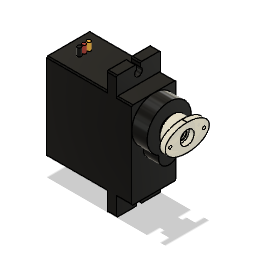
Door Assmebly (Autodesk Fusion 360 archive; units mm, degrees)
design "Micro Servo"
Autodesk Fusion 360 part; units mm, degrees
sketch "Sketch1" plane through (0, 0, 0) normal (0, 1, 0) x (1, 0, 0) in component "servo"
  line L0 (-0.0173, 0.0075) -> (22.1827, 0.0075)
  line L1 (22.1827, 0.0075) -> (22.1827, -12.1925)
  line L2 (22.1827, -12.1925) -> (-0.0173, -12.1925)
  line L3 (-0.0173, -12.1925) -> (-0.0173, 0.0075)
  line L4 (-0.0173, 0.0075) -> (22.1827, -12.1925) construction
  line L5 (22.1827, 0.0075) -> (-0.0173, -12.1925) construction
  point P0 (11.0827, -6.0925)
  dimension "d3" = 12.2
  dimension "d4" = 22.2
  constraint perpendicular L0 L1
  constraint parallel L0 L2
  constraint parallel L1 L3
  constraint horizontal L0
  constraint coincident L4 P0
  constraint coincident L5 P0
  measures "d3" distance of L0.end L1.end
  measures "d4" distance of L1.end L2.end
extrude "Extrude1" add sketch "Sketch1" along normal blind 22.62 in component "servo"
sketch "Sketch2" plane through (22.1827, 0, 0) normal (1, 0, 0) x (0, 0, -1) in component "servo"
  line L0 (-12.1925, 0) -> (0.0075, 0)
  line L1 (0.0075, 0) -> (0.0075, 22.62)
  line L2 (0.0075, 22.62) -> (-12.1925, 22.62)
  line L3 (-12.1925, 22.62) -> (-12.1925, 0)
  circle A0 centre (-5.7425, 16.87) radius 5.75
  dimension "d7" = 11.5
  constraint tangent L1 A0
  constraint tangent L2 A0
  measures "d7" diameter of A0
move_face "OffsetFaces1" offset -0.7 1 faces at (14.7827, 7.54, 12.1925) in component "servo"
extrude "Extrude2" add sketch "Sketch2" along normal blind 4 contours A0 in component "servo"
sketch "Sketch3" plane through (22.1827, 0, 0) normal (1, 0, 0) x (0, 0, -1) in component "servo"
  arc A0 (-11.4925, 16.87) -> (0.0075, 16.87) centre (-5.7425, 16.87) ccw
  line L0 (-11.4925, 16.87) -> (-11.4925, 0)
  line L1 (-11.4925, 0) -> (0.0075, 0)
  line L2 (0.0075, 0) -> (0.0075, 16.87)
  circle A1 centre (-5.7425, 11.12) radius 2.75
  dimension "d11" = 5.5
  constraint midpoint A0 A1.centre
  measures "d11" diameter of A1
extrude "Extrude3" add sketch "Sketch3" along normal blind 4 contours A0 A1 picked at (-5.7857, 10.2135) in component "servo"
sketch "Sketch4" plane through (26.1827, 0, 0) normal (1, 0, 0) x (0, 0, -1) in component "servo"
  arc A0 (-3.0723, 11.7776) -> (-8.4127, 11.7776) centre (-5.7425, 16.87) ccw
  arc A1 (-8.4127, 11.7776) -> (-3.0723, 11.7776) centre (-5.7425, 11.12) ccw
  circle A2 centre (-5.7425, 16.87) radius 2.4
  dimension "d14" = 4.8
  constraint concentric A0 A2
  measures "d14" diameter of A2
extrude "Extrude4" add sketch "Sketch4" along normal blind 3 contours A2 in component "servo"
sketch "Sketch5" plane through (0, 22.62, 0) normal (0, 1, 0) x (-1, 0, 0) in component "servo"
  line L0 (0.0173, 11.4925) -> (-22.1827, 11.4925)
  line L1 (-22.1827, 11.4925) -> (-22.1827, 5.7425)
  line L2 (-22.1827, 5.7425) -> (-22.1827, -0.0075)
  line L3 (-22.1827, -0.0075) -> (0.0173, -0.0075)
  line L4 (0.0173, -0.0075) -> (0.0173, 11.4925)
  line L5 (-18.1827, 0) -> (-15.7827, 0)
  line L6 (-15.7827, 0) -> (-15.7827, 11.485)
  line L7 (-15.7827, 11.485) -> (-18.1827, 11.485)
  line L8 (-18.1827, 11.485) -> (-18.1827, 0)
  line L9 (-18.1827, 0) -> (-15.7827, 11.485) construction
  line L10 (-15.7827, 0) -> (-18.1827, 11.485) construction
  line L11 (-22.1827, 11.4925) -> (0.0173, 11.4925)
  line L12 (0.0173, 11.4925) -> (0.0173, -0.0075)
  line L13 (0.0173, -0.0075) -> (-22.1827, -0.0075)
  line L14 (-22.1827, -0.0075) -> (-22.1827, 11.4925)
  point P0 (-16.9827, 5.7425)
  dimension "d17" = 2.4
  dimension "d18" = 4
  constraint perpendicular L5 L6
  constraint parallel L5 L7
  constraint parallel L6 L8
  constraint horizontal L5
  constraint coincident L9 P0
  constraint coincident L10 P0
  measures "d17" distance of L6.end L7.end
  measures "d18" distance of L1.end L8
extrude "Extrude5" add sketch "Sketch5" along normal blind 4.7 contours L5 L6 L7 L8 in component "servo"
sketch "Sketch6" plane through (0, 27.32, 0) normal (0, 1, 0) x (-1, 0, 0) in component "servo"
  line L0 (-18.1827, 11.485) -> (-18.1827, 0)
  line L1 (-18.1827, 0) -> (-15.7827, 0)
  line L2 (-15.7827, 0) -> (-15.7827, 11.485)
  line L3 (-15.7827, 11.485) -> (-18.1827, 11.485)
  line L4 (-22.1827, 11.4925) -> (0.0173, 11.4925)
  line L5 (0.0173, 11.4925) -> (0.0173, -0.0075)
  line L6 (0.0173, -0.0075) -> (-22.1827, -0.0075)
  line L7 (-22.1827, -0.0075) -> (-22.1827, 11.4925)
  line L8 (-22.1827, -0.0075) -> (0.0173, -0.0075)
  line L9 (0.0173, -0.0075) -> (-22.1827, -0.0075)
  line L10 (-15.7827, 11.485) -> (-18.1827, 11.485)
  line L11 (-18.1827, 11.485) -> (-15.7827, 11.485)
  line L12 (-18.1827, 0) -> (-15.7827, 0)
  line L13 (-15.7827, 0) -> (-18.1827, 0)
sketch "Sketch7" plane through (0, 0, 0) normal (0, -1, 0) x (1, 0, 0) in component "servo"
  line L0 (22.1827, 11.4925) -> (-0.0173, 11.4925)
  line L1 (-0.0173, 11.4925) -> (-0.0173, -0.0075)
  line L2 (-0.0173, -0.0075) -> (22.1827, -0.0075)
  line L3 (22.1827, -0.0075) -> (22.1827, 11.4925)
  line L4 (18.1827, 0) -> (15.7827, 0)
  line L5 (15.7827, 0) -> (15.7827, 11.485)
  line L6 (15.7827, 11.485) -> (18.1827, 11.485)
  line L7 (18.1827, 11.485) -> (18.1827, 0)
  line L8 (18.1827, 0) -> (15.7827, 11.485) construction
  line L9 (15.7827, 0) -> (18.1827, 11.485) construction
  point P0 (16.9827, 5.7425)
  point P1 (16.9827, 5.7425)
  point P2 (18.1827, 0)
  constraint perpendicular L4 L5
  constraint parallel L4 L6
  constraint parallel L5 L7
  constraint horizontal L4
  constraint coincident P2 L4.start
  constraint coincident L8 P1
  constraint coincident L9 P1
  constraint coincident P1 P0
extrude "Extrude6" add sketch "Sketch7" along normal blind 4.7 contours L4 L5 L6 L7 in component "servo"
sketch "Sketch8" plane through (18.1827, 0, 0) normal (1, 0, 0) x (0, 0, -1) in component "servo"
  line L0 (-11.485, 22.62) -> (0, 22.62)
  line L1 (0, 22.62) -> (0, 27.32)
  line L2 (0, 27.32) -> (-11.485, 27.32)
  line L3 (-11.485, 27.32) -> (-11.485, 22.62)
  circle A0 centre (-5.7425, 25.32) radius 1
  line L4 (-5.7425, 27.32) -> (-5.7425, 22.62) construction
  line L5 (-5.2425, 27.32) -> (-5.2425, 26.186)
  line L6 (-6.2425, 27.32) -> (-6.2425, 26.186)
  point P0 (-5.7425, 22.62)
  dimension "d23" = 2
  dimension "d24" = 2
  dimension "d27" = 1
  constraint midpoint L2 L4.start
  constraint coincident P0 L4.end
  constraint coincident A0.centre L4
  constraint coincident L2 L5.start
  constraint coincident A0 L5.end
  constraint perpendicular L2 L5
  constraint coincident L2 L6.start
  constraint coincident A0 L6.end
  constraint perpendicular L2 L6
  measures "d23" diameter of A0
  measures "d24" distance of L2 A0.centre
  measures "d27" distance of L5 L6
extrude "Extrude7" cut sketch "Sketch8" against normal up to surface (2.4 mm away) contours L2 A0 L5 L6 | A0 in component "servo"
sketch "Sketch9" plane through (18.1827, 0, 0) normal (1, 0, 0) x (0, 0, -1) in component "servo"
  line L0 (0, 0) -> (-11.485, 0)
  line L1 (-11.485, 0) -> (-11.485, -4.7)
  line L2 (-11.485, -4.7) -> (0, -4.7)
  line L3 (0, -4.7) -> (0, 0)
  circle A0 centre (-5.7412, -2.7) radius 1
  line L4 (-5.7425, 0) -> (-5.7425, -4.7) construction
  line L5 (-5.2425, -3.5668) -> (-5.2425, -4.7)
  line L6 (-6.2425, -3.5653) -> (-6.2425, -4.7)
  dimension "d30" = 2
  dimension "d31" = 2
  dimension "d33" = 1
  constraint midpoint L0 L4.start
  constraint midpoint L2 L4.end
  constraint coincident A0 L5.start
  constraint coincident L2 L5.end
  constraint perpendicular L2 L5
  constraint coincident A0 L6.start
  constraint coincident L2 L6.end
  constraint perpendicular L2 L6
  measures "d30" diameter of A0
  measures "d31" distance of A0.centre L4.end
  measures "d33" distance of L5 L6
extrude "Extrude8" cut sketch "Sketch9" against normal up to surface (2.4 mm away) contours L2 A0 L5 L6 | A0 in component "servo"
sketch "Sketch10" plane through (0, 0, -0.0075) normal (0, 0, -1) x (-1, 0, 0) in component "servo"
  line L0 (-22.1827, 0) -> (0.0173, 0)
  line L1 (0.0173, 0) -> (0.0173, 22.62)
  line L2 (0.0173, 22.62) -> (-22.1827, 22.62)
  line L3 (-22.1827, 22.62) -> (-22.1827, 16.87)
  line L4 (-22.1827, 16.87) -> (-22.1827, 0)
sketch "Sketch11" plane through (0, 22.62, 0) normal (0, 1, 0) x (-1, 0, 0) in component "servo"
  line L0 (-18.1827, 11.485) -> (-15.7827, 11.485)
  line L1 (-15.7827, 11.485) -> (-15.7827, 0)
  line L2 (-15.7827, 0) -> (-18.1827, 0)
  line L3 (-18.1827, 0) -> (-18.1827, 11.485)
  line L4 (0.0173, 11.4925) -> (-22.1827, 11.4925)
  line L5 (-22.1827, 11.4925) -> (-22.1827, 5.7425)
  line L6 (-22.1827, 5.7425) -> (-22.1827, -0.0075)
  line L7 (-22.1827, -0.0075) -> (0.0173, -0.0075)
  line L8 (0.0173, -0.0075) -> (0.0173, 11.4925)
  line L9 (-3.9827, 4.4925, 0) -> (-3.9827, 4.4925, 2)
  line L10 (0.0173, -0.0075) -> (-22.1827, -0.0075)
  line L11 (-3.9827, 5.7425, 0) -> (-3.9827, 5.7425, 2)
  line L12 (-3.9827, 6.9925, 0) -> (-3.9827, 6.9925, 2)
  dimension "d37" = 4
  dimension "d38" = 4.5
  dimension "d39" = 4.5
pipe "Pipe1" add diameter 1 path "Sketch11" along L9 in component "servo"
pipe "Pipe2" add diameter 1 path "Sketch11" along L11 in component "servo"
pipe "Pipe3" add diameter 1 path "Sketch11" along L12 in component "servo"
sketch "Sketch12" plane through (29.1827, 0, 0) normal (1, 0, 0) x (0, 0, -1) in component "servo"
  circle A0 centre (-5.7425, 16.87) radius 2.4
  circle A1 centre (-5.7425, 16.87) radius 3.45
  dimension "d53" = 6.9
  constraint concentric A0 A1
  measures "d53" diameter of A1
extrude "Extrude9" add sketch "Sketch12" against normal blind 2 in component "servo"
move_face "OffsetFaces2" offset 1.72 1 faces at (29.1827, 16.0878, 6.0495) in component "servo"
sketch "Sketch13" plane through (30.9027, 0, 0) normal (1, 0, 0) x (0, 0, -1) in component "servo"
  circle A0 centre (-5.7425, 16.87) radius 3.45
  ellipse E0 centre (-5.7425, 16.87) end of major axis (0.0075, 16.87) minor radius 3.45
  line L0 (-11.4925, 16.87) -> (0.0075, 16.87)
  line L1 (-5.7425, 13.42) -> (-5.7425, 20.32)
  line L2 (0.0075, 0) -> (0.0075, 22.62)
  point P0 (0.0075, 16.87)
  constraint concentric A0 E0
  constraint perpendicular L0 L2
  constraint coincident E0 L0.start
  constraint coincident E0 P0
  constraint coincident E0 L1.start
  constraint coincident E0 L1.end
extrude "Extrude10" add sketch "Sketch13" against normal blind 1.4 contours A0 E0 L0 | A0 E0 L0 | A0 E0 L0 | A0 E0 L0 in component "servo"
sketch "Sketch14" plane through (30.9027, 0, 0) normal (1, 0, 0) x (0, 0, -1) in component "servo"
  arc A0 (-5.7573, 13.42) -> (-5.7276, 13.42) centre (-5.7425, 16.87) ccw
  ellipse E0 centre (-5.7425, 16.87) end of major axis (0.0075, 16.87) minor radius 3.45 (-5.7276, 13.42) -> (-5.7276, 20.32) ccw
  arc A1 (-5.7276, 20.32) -> (-5.7573, 20.32) centre (-5.7425, 16.87) ccw
  ellipse E1 centre (-5.7425, 16.87) end of major axis (0.0075, 16.87) minor radius 3.45 (-5.7573, 20.32) -> (-5.7573, 13.42) ccw
  circle A2 centre (-1.3212, 16.87) radius 0.4
  circle A3 centre (-10.1636, 16.9081) radius 0.4
  line L0 (-5.7276, 20.32) -> (-5.7573, 13.42) construction
  dimension "d59" = 0.8
  dimension "d60" = 0.8
  constraint coincident A1.start L0.start
  constraint coincident A0.start L0.end
  constraint symmetric A2.centre A3.centre L0
  measures "d59" diameter of A2
  measures "d60" diameter of A3
extrude "Extrude11" cut sketch "Sketch14" against normal up to surface (1.4 mm away) contours A2 in component "servo"
extrude "Extrude12" cut sketch "Sketch14" against normal up to surface (1.4 mm away) contours A3 in component "servo"
sketch "Sketch15" plane through (30.9027, 0, 0) normal (1, 0, 0) x (0, 0, -1) in component "servo"
  circle A0 centre (-10.1636, 16.9081) radius 0.4
  circle A1 centre (-1.3212, 16.87) radius 0.4
  arc A2 (-5.7573, 13.42) -> (-5.7276, 13.42) centre (-5.7425, 16.87) ccw
  ellipse E0 centre (-5.7425, 16.87) end of major axis (0.0075, 16.87) minor radius 3.45 (-5.7276, 13.42) -> (-5.7276, 20.32) ccw
  arc A3 (-5.7276, 20.32) -> (-5.7573, 20.32) centre (-5.7425, 16.87) ccw
  ellipse E1 centre (-5.7425, 16.87) end of major axis (0.0075, 16.87) minor radius 3.45 (-5.7573, 20.32) -> (-5.7573, 13.42) ccw
  circle A4 centre (-5.7425, 16.87) radius 1.8
  dimension "d65" = 3.6
  constraint concentric A2 A4
  measures "d65" diameter of A4
extrude "Extrude13" cut sketch "Sketch15" against normal blind 1.3 contours A4 in component "servo"
sketch "Sketch16" plane through (29.6027, 0, 0) normal (1, 0, 0) x (0, 0, -1) in component "servo"
  circle A0 centre (-5.7425, 16.87) radius 1.8
  circle A1 centre (-5.7425, 16.87) radius 1.225
  dimension "d68" = 2.45
  constraint concentric A0 A1
  measures "d68" diameter of A1
extrude "Extrude14" cut sketch "Sketch16" against normal blind 0.2 contours A1 in component "servo"
sketch "Sketch17" plane through (29.4027, 0, 0) normal (1, 0, 0) x (0, 0, -1) in component "servo"
  circle A0 centre (-5.7425, 16.87) radius 1.225
  circle A1 centre (-5.7425, 16.87) radius 0.85
  dimension "d71" = 1.7
  constraint concentric A0 A1
  measures "d71" diameter of A1
extrude "Extrude15" cut sketch "Sketch17" against normal blind 3 contours A1 in component "servo"
thread "Thread1" "ISO Metric profile 1.6 M1.6x0.35 6H" major diameter 1.668 minor diameter 1.271 pitch 0.35 angle 60 resizes the face on face at (27.4027, 17.2002, 4.9592) in component "servo"
extrude "Extrude16" add 1 faces at (17.3827, -1.5667, 0) along direction (0, 0, -1) up to surface (0.0075 mm away) in component "servo"
extrude "Extrude17" add 1 faces at (16.5827, -1.5667, 11.485) along direction (0, 0, 1) up to surface (0.0075 mm away) in component "servo"
extrude "Extrude18" add 1 faces at (16.5827, 24.1867, 11.485) along direction (0, 0, 1) up to surface (0.0075 mm away) in component "servo"
extrude "Extrude19" add 1 faces at (17.3827, 24.1867, 0) along direction (0, 0, -1) up to surface (0.0075 mm away) in component "servo"
fillet "Fillet1" radius 0.3 16 edges at (7.8827, 22.62, -0.0075) (16.9827, 27.32, -0.0075) (16.9827, 27.32, 5.2425) (16.9827, 27.32, 6.2425) (16.9827, 27.32, 11.4925) (20.1827, 22.62, 11.4925) (20.1827, 22.62, -0.0075) (7.8827, 22.62, 11.4925) (20.1827, 0, -0.0075) (7.8827, 0, -0.0075) (16.9827, -4.7, -0.0075) (16.9827, -4.7, 6.2425) (16.9827, -4.7, 5.2425) (16.9827, -4.7, 11.4925) (20.1827, 0, 11.4925) (7.8827, 0, 11.4925) in component "servo"
component "servo" placed x (1, 0, 0) y (0, 1, 0) z (0, 0, 1) at (0, 0, 0)

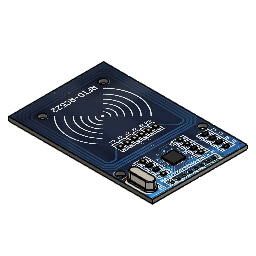
design "RFID"
Autodesk Fusion 360 part; units mm, degrees
sketch "Sketch1" plane through (0, 0, 0) normal (0, 1, 0) x (1, 0, 0) in component "Base"
  line L0 (0, 0) -> (60, 0)
  line L1 (60, 0) -> (60, -39.6)
  line L2 (60, -39.6) -> (0, -39.6)
  line L3 (0, -39.6) -> (0, 0)
  circle A0 centre (7.05, -32.45) radius 1.55
  line L4 (5.5, -34) -> (0, -34) construction
  line L5 (5.5, -34) -> (5.5, -39.6) construction
  circle A1 centre (7.05, -7.15) radius 1.55
  line L6 (5.5, 0) -> (5.5, -5.6) construction
  line L7 (5.5, -5.6) -> (0, -5.6) construction
  line L8 (0, -1.0831) -> (42.4499, -1) construction
  line L9 (42.4499, -1) -> (42.4499, 0) construction
  circle A2 centre (43.9999, -2.547) radius 1.55
  line L10 (0, -38.6) -> (42.45, -38.6) construction
  line L11 (42.45, -38.6) -> (42.45, -39.6) construction
  circle A3 centre (44, -37.05) radius 1.55
  line L12 (49.05, -33.9) -> (55.45, -33.9)
  line L13 (57.6, -36.05) -> (57.6, -36.15)
  line L14 (55.45, -38.3) -> (49.05, -38.3)
  line L15 (46.9, -36.15) -> (46.9, -36.05)
  arc A4 (49.05, -33.9) -> (46.9, -36.05) centre (49.05, -36.05) ccw
  arc A5 (46.9, -36.15) -> (49.05, -38.3) centre (49.05, -36.15) ccw
  arc A6 (57.6, -36.05) -> (55.45, -33.9) centre (55.45, -36.05) ccw
  arc A7 (55.45, -38.3) -> (57.6, -36.15) centre (55.45, -36.15) ccw
  line L16 (55.45, -37.85) -> (49.05, -37.85)
  arc A8 (47.35, -36.15) -> (49.05, -37.85) centre (49.05, -36.15) ccw
  line L17 (47.35, -36.15) -> (47.35, -36.05)
  arc A9 (49.05, -34.35) -> (47.35, -36.05) centre (49.05, -36.05) ccw
  line L18 (49.05, -34.35) -> (55.45, -34.35)
  arc A10 (57.15, -36.05) -> (55.45, -34.35) centre (55.45, -36.05) ccw
  line L19 (57.15, -36.05) -> (57.15, -36.15)
  arc A11 (55.45, -37.85) -> (57.15, -36.15) centre (55.45, -36.15) ccw
  line L20 (46.9, -38.3) -> (46.9, -39.6) construction
  line L21 (57.6, -33.9) -> (60, -33.9) construction
  line L22 (58, -39.6) -> (58, -29.2) construction
  line L23 (58, -29.2) -> (60, -29.2) construction
  circle A12 centre (58, -29.2) radius 0.525
  circle A13 centre (58, -26.7) radius 0.525
  circle A14 centre (58, -24.2) radius 0.525
  circle A15 centre (58, -21.7) radius 0.525
  circle A16 centre (58, -19.2) radius 0.525
  circle A17 centre (58, -16.7) radius 0.525
  circle A18 centre (58, -14.2) radius 0.525
  circle A19 centre (58, -11.7) radius 0.525
  point P0 (46.9, -33.9)
  point P1 (57.6, -33.9)
  point P2 (46.9, -38.3)
  dimension "d1" = 60
  dimension "d2" = 39.6
  dimension "d5" = 3.1
  dimension "d8" = 5.6
  dimension "d9" = 5.5
  dimension "d10" = 3.1
  dimension "d11" = 5.6
  dimension "d12" = 5.5
  dimension "d13" = 42.45
  dimension "d14" = 1
  dimension "d15" = 3.1
  dimension "d16" = 42.45
  dimension "d17" = 1
  dimension "d18" = 3.1
  dimension "d19" = 10.7
  dimension "d20" = 4.4
  dimension "d23" = 0.45
  dimension "d24" = 2.15
  dimension "d25" = 2.4
  dimension "d26" = 1.3
  dimension "d27" = 10.4
  dimension "d28" = 2
  dimension "d29" = 1.05
  dimension "d32" = 0
  dimension "d33" = 2.5
  constraint horizontal L0
  constraint vertical L1
  constraint horizontal L2
  constraint vertical L3
  constraint coincident L0.start L3.end
  constraint coincident L3 L4.end
  constraint perpendicular L3 L4
  constraint coincident L2 L5.end
  constraint perpendicular L2 L5
  constraint coincident L0 L6.start
  constraint tangent A1 L6
  constraint coincident L3 L7.end
  constraint perpendicular L3 L7
  constraint tangent A1 L7
  constraint coincident L3 L8.start
  constraint coincident L0 L9.end
  constraint perpendicular L0 L9
  constraint tangent L8 A2
  constraint tangent L9 A2
  constraint coincident L3 L10.start
  constraint coincident L2 L11.end
  constraint perpendicular L2 L11
  constraint tangent L11 A3
  constraint tangent L10 A3
  constraint coincident P0 L12
  constraint coincident P0 L15
  constraint tangent L12 A4
  constraint tangent L15 A4
  constraint coincident P2 L14
  constraint coincident P2 L15
  constraint tangent L14 A5
  constraint tangent L15 A5
  constraint equal A4 A5
  constraint coincident P1 L12
  constraint coincident P1 L13
  constraint tangent L12 A6
  constraint tangent L13 A6
  constraint equal A4 A6
  constraint tangent L13 A7
  constraint tangent L14 A7
  constraint equal A4 A7
  constraint coincident P2 L20.start
  constraint coincident L2 L20.end
  constraint perpendicular L2 L20
  constraint coincident P1 L21.start
  constraint coincident L1 L21.end
  constraint perpendicular L1 L21
  constraint coincident L2 L22.start
  constraint coincident L1 L23.end
  constraint perpendicular L1 L23
  constraint coincident L22.end L23.start
  measures "d1" distance of L0.start L0.end
  measures "d2" distance of L0.start L2.end
  measures "d5" diameter of A0
  measures "d8" distance of L4.start L5.end
  measures "d9" distance of L4.start L4.end
  measures "d10" diameter of A1
  measures "d11" distance of L6.start L6.end
  measures "d12" distance of L6.end L7.end
  measures "d13" distance of L8.start L8.end
  measures "d14" distance of L8.end L9.end
  measures "d15" diameter of A2
  measures "d16" distance of L10.start L10.end
  measures "d17" distance of L10.end L11.end
  measures "d18" diameter of A3
  measures "d19" distance of P0 P1
  measures "d20" distance of P0 P2
  measures "d24" radius of A4
  measures "d25" distance of P1 L21.end
  measures "d26" distance of P2 L20.end
  measures "d27" distance of L22.start L22.end
  measures "d28" distance of L22.end L23.end
  measures "d29" diameter of A12
extrude "Extrude1" add sketch "Sketch1" against normal blind 1.6 contours L0 L1 L2 L3 | L12 L13 L14 L15 A4 A5 A6 A7 | L16 A8 L17 A9 L18 A10 L19 A11 makes body 1 in component "Base"
extrude "Extrude2" add sketch "Sketch1" along normal blind 0.7 separate body contours L12 L13 L14 L15 A4 A5 A6 A7 | L16 A8 L17 A9 L18 A10 L19 A11 makes body 2 in component "Base"
extrude "Extrude3" add sketch "Sketch1" along normal blind 3.55 separate body contours L16 A8 L17 A9 L18 A10 L19 A11 makes body 3 in component "Base"
fillet "Fillet1" radius 0.25 8 edges at (47.35, 3.55, 36.1) (47.8479, 3.55, 37.3521) (52.25, 3.55, 37.85) (56.6521, 3.55, 37.3521) (57.15, 3.55, 36.1) (56.6521, 3.55, 34.8479) (52.25, 3.55, 34.35) (47.8479, 3.55, 34.8479) on bodies 3 in component "Base"
combine "Combine1" operation add target body 2 tool bodies 3 in component "Base"
sketch "Sketch2" plane through (0, 0, 0) normal (0, 1, 0) x (1, 0, 0) in component "Base"
  line L0 (47.0522, -4.3477) -> (48.2693, -4.3477)
  line L1 (48.2693, -4.3477) -> (48.2693, -6.0785)
  line L2 (48.2693, -6.0785) -> (47.0522, -6.0785)
  line L3 (47.0522, -6.0785) -> (47.0522, -4.3477)
  line L4 (49.9732, -4.226) -> (51.1904, -4.226)
  line L5 (51.1904, -4.226) -> (51.1904, -5.9568)
  line L6 (51.1904, -5.9568) -> (49.9732, -5.9568)
  line L7 (49.9732, -5.9568) -> (49.9732, -4.226)
  line L8 (52.7686, -4.3029) -> (53.9858, -4.3029)
  line L9 (53.9858, -4.3029) -> (53.9858, -6.0337)
  line L10 (53.9858, -6.0337) -> (52.7686, -6.0337)
  line L11 (52.7686, -6.0337) -> (52.7686, -4.3029)
  line L12 (55.7501, -4.3253) -> (56.9673, -4.3253)
  line L13 (56.9673, -4.3253) -> (56.9673, -6.0561)
  line L14 (56.9673, -6.0561) -> (55.7501, -6.0561)
  line L15 (55.7501, -6.0561) -> (55.7501, -4.3253)
  line L16 (43.8016, -11.8351) -> (45.0188, -11.8351)
  line L17 (45.0188, -11.8351) -> (45.0188, -13.0727)
  line L18 (45.0188, -13.0727) -> (43.8016, -13.0727)
  line L19 (43.8016, -13.0727) -> (43.8016, -11.8351)
  line L20 (46.8056, -11.8576) -> (48.0227, -11.8576)
  line L21 (48.0227, -11.8576) -> (48.0227, -13.0951)
  line L22 (48.0227, -13.0951) -> (46.8056, -13.0951)
  line L23 (46.8056, -13.0951) -> (46.8056, -11.8576)
  line L24 (43.8016, -11.8351) -> (45.0188, -11.8351)
  line L25 (45.0188, -11.8351) -> (45.0188, -13.0727)
  line L26 (45.0188, -13.0727) -> (43.8016, -13.0727)
  line L27 (43.8016, -13.0727) -> (43.8016, -11.8351)
  line L28 (49.675, -11.7006) -> (50.8922, -11.7006)
  line L29 (50.8922, -11.7006) -> (50.8922, -13.4314)
  line L30 (50.8922, -13.4314) -> (49.675, -13.4314)
  line L31 (49.675, -13.4314) -> (49.675, -11.7006)
  line L32 (52.5668, -11.9024) -> (53.784, -11.9024)
  line L33 (53.784, -11.9024) -> (53.784, -13.14)
  line L34 (53.784, -13.14) -> (52.5668, -13.14)
  line L35 (52.5668, -13.14) -> (52.5668, -11.9024)
  line L36 (46.8596, -17.6793) -> (52.06, -17.6793)
  line L37 (52.06, -17.6793) -> (52.06, -22.8023)
  line L38 (52.06, -22.8023) -> (46.8596, -22.8023)
  line L39 (46.8596, -22.8023) -> (46.8596, -17.6793)
  line L40 (33.7509, -12.0901) -> (35.1413, -12.0901)
  line L41 (35.1413, -12.0901) -> (35.1413, -13.3759)
  line L42 (35.1413, -13.3759) -> (33.7509, -13.3759)
  line L43 (33.7509, -13.3759) -> (33.7509, -12.0901)
  line L44 (33.736, -15.0653) -> (35.1264, -15.0653)
  line L45 (33.736, -16.3511) -> (33.736, -15.0653)
  line L46 (35.1264, -15.0653) -> (35.1264, -16.3511)
  line L47 (35.1264, -16.3511) -> (33.736, -16.3511)
  line L48 (33.6911, -17.9209) -> (35.0815, -17.9209)
  line L49 (33.6911, -19.2067) -> (33.6911, -17.9209)
  line L50 (35.0815, -17.9209) -> (35.0815, -19.2067)
  line L51 (35.0815, -19.2067) -> (33.6911, -19.2067)
  line L52 (33.6691, -20.8381) -> (35.0596, -20.8381)
  line L53 (33.6691, -22.1239) -> (33.6691, -20.8381)
  line L54 (35.0596, -20.8381) -> (35.0596, -22.1239)
  line L55 (35.0596, -22.1239) -> (33.6691, -22.1239)
  line L56 (33.7108, -23.8497) -> (35.1012, -23.8497)
  line L57 (33.7108, -25.1354) -> (33.7108, -23.8497)
  line L58 (35.1012, -23.8497) -> (35.1012, -25.1354)
  line L59 (35.1012, -25.1354) -> (33.7108, -25.1354)
  line L60 (33.7803, -26.782) -> (35.1708, -26.782)
  line L61 (33.7803, -28.0678) -> (33.7803, -26.782)
  line L62 (35.1708, -26.782) -> (35.1708, -28.0678)
  line L63 (35.1708, -28.0678) -> (33.7803, -28.0678)
  line L64 (43.9054, -27.4668) -> (45.1225, -27.4668)
  line L65 (45.1225, -27.4668) -> (45.1225, -28.7044)
  line L66 (45.1225, -28.7044) -> (43.9054, -28.7044)
  line L67 (43.9054, -28.7044) -> (43.9054, -27.4668)
  line L68 (43.8016, -11.8351) -> (45.0188, -11.8351)
  line L69 (45.0188, -11.8351) -> (45.0188, -13.0727)
  line L70 (45.0188, -13.0727) -> (43.8016, -13.0727)
  line L71 (43.8016, -13.0727) -> (43.8016, -11.8351)
  line L72 (52.5824, -27.5841) -> (53.7996, -27.5841)
  line L73 (53.7996, -27.5841) -> (53.7996, -28.8217)
  line L74 (53.7996, -28.8217) -> (52.5824, -28.8217)
  line L75 (52.5824, -28.8217) -> (52.5824, -27.5841)
  line L76 (46.643, -27.2525) -> (47.8602, -27.2525)
  line L77 (47.8602, -27.2525) -> (47.8602, -28.9833)
  line L78 (47.8602, -28.9833) -> (46.643, -28.9833)
  line L79 (46.643, -28.9833) -> (46.643, -27.2525)
  line L80 (49.5422, -27.2928) -> (50.7594, -27.2928)
  line L81 (50.7594, -27.2928) -> (50.7594, -29.0236)
  line L82 (50.7594, -29.0236) -> (49.5422, -29.0236)
  line L83 (49.5422, -29.0236) -> (49.5422, -27.2928)
  constraint horizontal L0
  constraint vertical L1
  constraint horizontal L2
  constraint vertical L3
  constraint horizontal L4
  constraint vertical L5
  constraint horizontal L6
  constraint vertical L7
  constraint horizontal L8
  constraint vertical L9
  constraint horizontal L10
  constraint vertical L11
  constraint horizontal L12
  constraint vertical L13
  constraint horizontal L14
  constraint vertical L15
  constraint horizontal L16
  constraint vertical L17
  constraint horizontal L18
  constraint vertical L19
  constraint horizontal L20
  constraint vertical L21
  constraint horizontal L22
  constraint vertical L23
  constraint horizontal L24
  constraint vertical L25
  constraint horizontal L26
  constraint vertical L27
  constraint horizontal L28
  constraint vertical L29
  constraint horizontal L30
  constraint vertical L31
  constraint horizontal L32
  constraint vertical L33
  constraint horizontal L34
  constraint vertical L35
  constraint horizontal L36
  constraint vertical L37
  constraint horizontal L38
  constraint vertical L39
  constraint horizontal L40
  constraint vertical L41
  constraint horizontal L42
  constraint vertical L43
  constraint horizontal L44
  constraint vertical L46
  constraint horizontal L47
  constraint vertical L45
  constraint horizontal L48
  constraint vertical L50
  constraint horizontal L51
  constraint vertical L49
  constraint horizontal L52
  constraint vertical L54
  constraint horizontal L55
  constraint vertical L53
  constraint horizontal L56
  constraint vertical L58
  constraint horizontal L59
  constraint vertical L57
  constraint horizontal L60
  constraint vertical L62
  constraint horizontal L63
  constraint vertical L61
  constraint horizontal L64
  constraint vertical L65
  constraint horizontal L66
  constraint vertical L67
  constraint horizontal L68
  constraint vertical L69
  constraint horizontal L70
  constraint vertical L71
  constraint horizontal L72
  constraint vertical L73
  constraint horizontal L74
  constraint vertical L75
  constraint horizontal L76
  constraint vertical L77
  constraint horizontal L78
  constraint vertical L79
  constraint horizontal L80
  constraint vertical L81
  constraint horizontal L82
  constraint vertical L83
extrude "Extrude4" add sketch "Sketch2" along normal blind 0.5 separate body makes body 4 at (49.948, 0, 28.4466) makes body 5 at (50.0807, 0, 12.2776) makes body 6 at (34.6378, 0, 24.7069) makes body 7 at (34.2144, 0, 12.5187) makes body 8 at (50.379, 0, 5.3799) makes body 9 at (56.1558, 0, 4.9022) makes body 10 at (34.1326, 0, 21.2667) makes body 11 at (47.2113, 0, 12.6826) makes body 12 at (47.0487, 0, 28.4064) makes body 13 at (52.9881, 0, 27.9966) makes body 14 at (52.9726, 0, 12.3149) makes body 15 at (34.2438, 0, 27.2106) makes body 16 at (34.1994, 0, 15.4939) makes body 17 at (47.8636, 0, 5.5016) makes body 18 at (53.1743, 0, 4.8798) makes body 19 at (34.1546, 0, 18.3495) makes body 20 at (44.6131, 0, 12.2477) makes body 21 at (44.3111, 0, 28.2919) makes body 22 at (48.5931, 0, 19.3869) in component "Base"
component "Base" placed x (1, 0, 0) y (0, 1, 0) z (0, 0, 1) at (0, 0, 0)
component "Pins" placed x (1, 0, 0) y (0, 1, 0) z (0, 0, 1) at (0, 0, 0)
equation "d39 = 5.15 mm - 1.6 mm"
named bodies: "base", "Clock"
